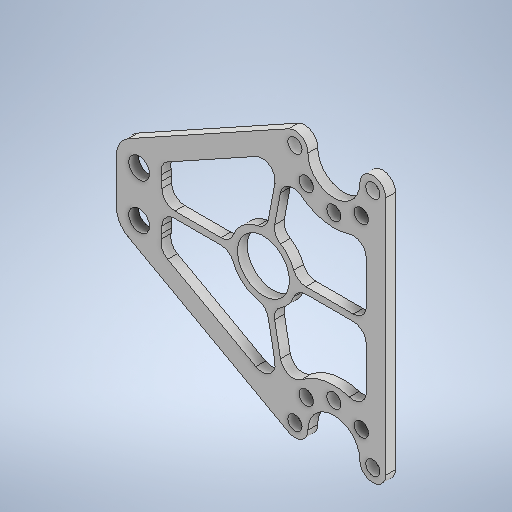
# Autodesk Inventor part: hiza
Saved by Autodesk Inventor 2025.1 (Build 291241000, 241)
## iProperties
Created: 2024-09-02
Part Number: hiza
Material: 一般
Document SubType Name: Modeling
Designer: right
Density: 1 g/cm^3
Appearance: 既定
Author: right
Autodesk Inventor part; units mm, degrees
ref_plane "YZ Plane" through (0, 0, 0) normal (1, 0, 0) x (0, 1, 0)
ref_plane "XZ Plane" through (0, 0, 0) normal (0, 1, 0) x (-1, 0, 0)
ref_plane "XY Plane" through (0, 0, 0) normal (0, 0, 1) x (1, 0, 0)
sketch "スケッチ1" plane through (0, 0, 0) normal (0, 0, 1) x (1, 0, 0)
  line L0 (5.096, 0) -> (-5.096, 0) construction
  circle A0 centre (20, 18.5) radius 4
  circle A1 centre (20, 18.5) radius 8
  circle A2 centre (20, 18.5) radius 6 construction
  circle A3 centre (20, 24.5) radius 1.1
  circle A4 centre (15.7574, 22.7426) radius 1.1
  circle A5 centre (14, 18.5) radius 1.1
  circle A6 centre (15.7574, 14.2574) radius 1.1
  circle A7 centre (20, 12.5) radius 1.1
  circle A8 centre (24.2426, 14.2574) radius 1.1
  circle A9 centre (26, 18.5) radius 1.1
  circle A10 centre (24.2426, 22.7426) radius 1.1
  circle A11 centre (-10, 3.5) radius 1.6
  circle A12 centre (20, -18.5) radius 4
  circle A13 centre (20, -18.5) radius 8
  circle A14 centre (20, -18.5) radius 6 construction
  circle A15 centre (20, -24.5) radius 1.1
  circle A16 centre (15.7574, -22.7426) radius 1.1
  circle A17 centre (14, -18.5) radius 1.1
  circle A18 centre (15.7574, -14.2574) radius 1.1
  circle A19 centre (20, -12.5) radius 1.1
  circle A20 centre (24.2426, -14.2574) radius 1.1
  circle A21 centre (26, -18.5) radius 1.1
  circle A22 centre (24.2426, -22.7426) radius 1.1
  circle A23 centre (-10, -3.5) radius 1.6
  circle A24 centre (-10, 3.5) radius 3.5
  circle A25 centre (-10, -3.5) radius 3.5
  line L1 (-11.6951, 6.5621) -> (13.0314, 20.2498)
  line L2 (28, 18.5) -> (28, -18.5)
  circle A26 centre (14, 18.5) radius 2
  circle A27 centre (26, 18.5) radius 2
  line L3 (-11.6951, -6.5621) -> (13.0314, -20.2498)
  circle A28 centre (14, -18.5) radius 2
  circle A29 centre (26, -18.5) radius 2
  line L4 (-13.5, 3.5) -> (-13.5, -3.5)
  point P0 (0, 0)
  point P1 (0, 0)
  point P2 (12.0954, 19.7317)
  point P3 (12.0954, -19.7317)
  point P4 (28, -18.5)
  point P5 (28, 18.5)
  point P6 (24, 18.5)
  point P7 (16, 18.5)
  point P8 (12.0954, -19.7317)
  point P9 (12, -18.5)
  point P10 (16, -18.5)
  point P11 (24, -18.5)
  dimension "d2" = 12
  dimension "d0" = 8
  dimension "d1" = 16
  dimension "d3" = 2.2
  dimension "d6" = 360
  dimension "d9" = 3.2
  dimension "d10" = 30
  dimension "d11" = 15
  dimension "d12" = 20
  dimension "d13" = 7
  constraints: 24 centre point, 17 symmetric about line, 10 end point, 8 coincident, 6 tangent, 4 point on circle, 3 horizontal, 3 vertical alignment, 2 midpoint, 2 point on line, 2 vertical, 47 other
  measures "d0" diameter of A0
  measures "d1" diameter of A1
  measures "d3" diameter of A3
  measures "d9" diameter of A11
  measures "d10" horizontal distance of A0.centre A11.centre
  measures "d11" vertical distance of A11.centre A0.centre
  measures "d12" horizontal distance of point (0, 0) A0.centre
  measures "d13" diameter of A24
extrude "押し出し1" add sketch "スケッチ1" along normal blind 1.5 contours A27 A1 A26 A0 | A27 | A26 | L2 A13 L3 A25 A24 L1 A1 | A26 A1 L1 | A29 A12 A28 A13 | A29 | A24 | A28 L3 A13 | A28 | A24 A25 L4 | A25
sketch "スケッチ2" plane through (0, 0, 1.5) normal (0, 0, 1) x (1, 0, 0)
  arc A0 (16, 18.5) -> (24, 18.5) centre (20, 18.5) ccw projected
  circle A1 centre (20, 18.5) radius 8
  arc A2 (24, -18.5) -> (16, -18.5) centre (20, -18.5) ccw projected
  arc A3 (24, -18.5) -> (28, -18.5) centre (26, -18.5) ccw projected
  circle A4 centre (20, -18.5) radius 8
  circle A5 centre (-10, 3.5) radius 1.6 projected
  circle A6 centre (-10, 3.5) radius 3.5
  circle A7 centre (-10, -3.5) radius 1.6 projected
  circle A8 centre (-10, -3.5) radius 3.5
  arc A9 (28, 18.5) -> (24, 18.5) centre (26, 18.5) ccw projected
  arc A10 (16, 18.5) -> (24, 18.5) centre (20, 18.5) ccw projected
  arc A11 (16, 18.5) -> (13.0314, 20.2498) centre (14, 18.5) ccw projected
  line L0 (13.0314, 20.2498) -> (-11.6951, 6.5621) projected
  arc A12 (-11.6951, 6.5621) -> (-13.5, 3.5) centre (-10, 3.5) ccw projected
  line L1 (-13.5, 3.5) -> (-13.5, -3.5) projected
  arc A13 (-13.5, -3.5) -> (-11.6951, -6.5621) centre (-10, -3.5) ccw projected
  line L2 (-11.6951, -6.5621) -> (13.0314, -20.2498) projected
  arc A14 (13.0314, -20.2498) -> (16, -18.5) centre (14, -18.5) ccw projected
  arc A15 (24, -18.5) -> (16, -18.5) centre (20, -18.5) ccw projected
  arc A16 (24, -18.5) -> (28, -18.5) centre (26, -18.5) ccw projected
  line L3 (28, -18.5) -> (28, 18.5) projected
  circle A17 centre (14, 18.5) radius 1.1 projected
  circle A18 centre (26, 18.5) radius 1.1 projected
  circle A19 centre (14, -18.5) radius 1.1 projected
  circle A20 centre (26, -18.5) radius 1.1 projected
  circle A21 centre (24.2426, -14.2574) radius 1.1 projected
  circle A22 centre (20, -12.5) radius 1.1 projected
  circle A23 centre (15.7574, -14.2574) radius 1.1 projected
  circle A24 centre (-10, -3.5) radius 1.6 projected
  circle A25 centre (-10, 3.5) radius 1.6 projected
  circle A26 centre (24.2426, 14.2574) radius 1.1 projected
  circle A27 centre (20, 12.5) radius 1.1 projected
  circle A28 centre (15.7574, 14.2574) radius 1.1 projected
  line L4 (-7.2114, 5.6151) -> (12.2793, 16.4045)
  line L5 (25, 12.255) -> (25, -12.255)
  line L6 (12.2793, -16.4045) -> (-7.2114, -5.6151)
  line L7 (-6.5, 3.5) -> (-6.5, -3.5)
  line L8 (-6.5, 0) -> (25, 0) construction
  line L9 (-6.5, 0.5) -> (25, 0.5)
  line L10 (-6.5, -0.5) -> (25, -0.5)
  line L11 (12.2793, 16.4045) -> (9.25, 0.5) construction
  line L12 (11.7103, 16.0895) -> (8.741, 0.5)
  line L13 (9.759, 0.5) -> (12.6058, 15.4462)
  line L14 (11.7103, -16.0895) -> (8.741, -0.5)
  line L15 (9.759, -0.5) -> (12.6058, -15.4462)
  line L16 (9.25, 0.5) -> (9.1548, 0) construction
  circle A29 centre (9.1548, 0) radius 4
  circle A30 centre (9.1548, 0) radius 5
  point P0 (0, 0)
  point P1 (-11.6951, 6.5621)
  point P2 (11.7103, -16.0895)
  point P3 (8.741, -0.5)
  point P4 (-6.5, -0.5)
  point P5 (9.759, -0.5)
  point P6 (12.6058, -15.4462)
  point P7 (10.5768, 4.7935)
  point P8 (14.1297, 0.5)
  point P9 (14.1297, -0.5)
  point P10 (10.5768, -4.7935)
  point P11 (9.5944, -4.9806)
  point P12 (4.1798, -0.5)
  point P13 (4.1798, 0.5)
  point P14 (9.5944, 4.9806)
  dimension "d16" = 3
  dimension "d17" = 3
  dimension "d18" = 3
  dimension "d19" = 0.5
  dimension "d20" = 0.5
  dimension "d21" = 0.5
  dimension "d25" = 8
  dimension "d26" = 10
  constraints: 26 end point, 12 point on circle, 6 centre point, 6 coincident, 6 point on line, 6 symmetric about line, 5 parallel, 3 midpoint, 3 tangent, 1 collinear
  measures "d16" distance between parallel lines of L0 L4
  measures "d17" distance between parallel lines of L3 L5
  measures "d18" distance between parallel lines of L2 L6
  measures "d19" distance between parallel lines of L8 L9
  measures "d20" distance between parallel lines of L11 L13
  measures "d21" distance between parallel lines of L12 L11
  measures "d25" diameter of A29
  measures "d26" diameter of A30
extrude "押し出し2" cut sketch "スケッチ2" against normal through all contours L5 L9 A30 L13 A1 | A4 L15 A30 L10 L5 | L12 A30 L9 L7 A6 L4 | A29 L9 L13 | L13 L9 L12 A29 | A29 L10 L9 | L6 A8 L7 L10 A30 L14 | L12 L9 A29 | A29 L15 L10 | A29 L14 L10 L15 | A29 L10 L14
fillet "フィレット1" radius 2 20 edges at (-7.2114, 5.6151, 0.75) (-6.5, 0.5, 0.75) (-6.5, -0.5, 0.75) (-7.2114, -5.6151, 0.75) (11.7103, -16.0895, 0.75) (12.6058, -15.4462, 0.75) (25, -12.255, 0.75) (25, 0.5, 0.75) (25, -0.5, 0.75) (25, 12.255, 0.75) (12.6058, 15.4462, 0.75) (11.7103, 16.0895, 0.75) (4.1798, -0.5, 0.75) (4.1798, 0.5, 0.75) (9.5944, 4.9806, 0.75) (10.5768, 4.7935, 0.75) (14.1297, 0.5, 0.75) (14.1297, -0.5, 0.75) (9.5944, -4.9806, 0.75) (10.5768, -4.7935, 0.75)
equation "\"d18\" = d16"
equation "\"d20\" = d21"
equation "\"d21\" = d19"
